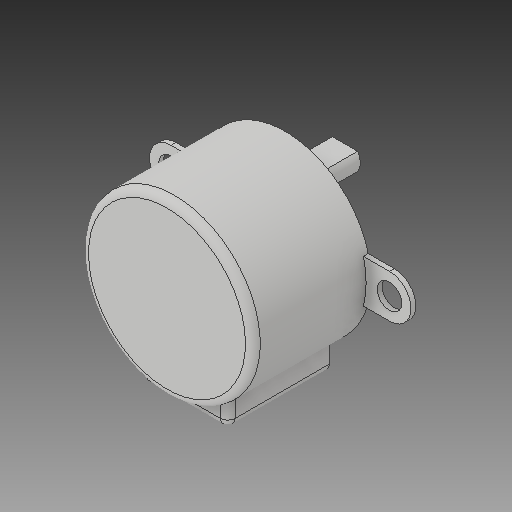
# Autodesk Inventor part: STEPPER MOTOR
Saved by Autodesk Inventor 2017 (Build 210142000, 142)
## iProperties
Created: 2017-04-01
Part Number: STEPPER MOTOR
Material: Generic
Document SubType Name: Modeling
Designer: Muchen
Density: 1 g/cm^3
Appearance: Default
Mass: 12.708 g
Surface Area: 34.3035 cm^2
Volume: 12.708 cm^3
Author: Muchen
Autodesk Inventor part; units mm, degrees
ref_plane "YZ Plane" through (0, 0, 0) normal (1, 0, 0) x (0, 1, 0)
ref_plane "XZ Plane" through (0, 0, 0) normal (0, 1, 0) x (-1, 0, 0)
ref_plane "XY Plane" through (0, 0, 0) normal (0, 0, 1) x (1, 0, 0)
sketch "Sketch1" plane through (0, 0, 0) normal (0, 0, 1) x (1, 0, 0)
  line L0 (0, 0) -> (0, 30.3704) construction
  line L1 (0, 0) -> (7.18, 0)
  line L2 (7.18, 0) -> (7.18, 4.46)
  arc A0 (0, 2.4704) -> (0, 30.3704) centre (0, 16.4204) ccw
  line L3 (13.5038, 19.9204) -> (17.75, 19.9204)
  arc A1 (17.75, 12.9204) -> (17.75, 19.9204) centre (17.75, 16.4204) ccw
  line L4 (17.75, 12.9204) -> (13.5038, 12.9204)
  circle A2 centre (17.75, 16.4204) radius 2
  line L5 (0, 0) -> (-7.18, 0)
  line L6 (-7.18, 0) -> (-7.18, 4.46)
  arc A3 (0, 30.3704) -> (0, 2.4704) centre (0, 16.4204) ccw
  line L7 (-13.5038, 19.9204) -> (-17.75, 19.9204)
  arc A4 (-17.75, 19.9204) -> (-17.75, 12.9204) centre (-17.75, 16.4204) ccw
  line L8 (-17.75, 12.9204) -> (-13.5038, 12.9204)
  circle A5 centre (-17.75, 16.4204) radius 2
  circle A6 centre (0, 22.2972) radius 4.61
  circle A7 centre (0, 22.2972) radius 2.5
  line L9 (2.0541, 23.7222) -> (-2.0541, 23.7222)
  line L10 (2.0541, 20.8722) -> (-2.0541, 20.8722)
  dimension "d0" = 13.95
  dimension "d1" = 7.18
  dimension "d2" = 4.46
  dimension "d3" = 3.5
  dimension "d4" = 4
  dimension "d11" = 9.22
  dimension "d12" = 5
  dimension "d13" = 2.85
  dimension "d26" = 35.5
  constraints: 22 end point, 18 point on circle, 8 centre point, 8 symmetric about line, 3 coincident, 3 parallel, 2 horizontal, 2 perpendicular, 2 point on line, 2 tangent, 1 horizontal alignment, 1 line through centre, 1 vertical, 3 other
  measures "d0" radius of A0
  measures "d1" distance of L0.start L1.end
  measures "d2" distance of L1.end L2.end
  measures "d3" radius of A1
  measures "d4" diameter of A2
  measures "d11" diameter of A6
  measures "d12" diameter of A7
  measures "d13" distance between parallel lines of L9 L10
  measures "d26" distance of A4.centre A2.centre
extrude "Extrusion1" add sketch "Sketch1" along normal blind 19.2 contours A0 A3 | A6 | A7 L10 L9 | L9 A7 | A7 L10
extrude "Extrusion2" add sketch "Sketch1" along normal blind 0.79 contours A0 L3 A1 L4 | L8 A4 L7 A3
extrude "Extrusion3" add sketch "Sketch1" along normal blind 16.5 contours L5 L6 A3 A0 L2 L1
extrude "Extrusion4" add sketch "Sketch1" against normal blind 1.75 contours A6
extrude "Extrusion5" add sketch "Sketch1" against normal blind 3.78 contours L9 A7 | A7 L10
extrude "Extrusion6" add sketch "Sketch1" against normal blind 9.73 contours A7 L10 L9
fillet "Fillet1" radius 1.2 6 edges at (7.18, 28.3807, 19.2) (7.18, 0, 8.25) (0, 0, 16.5) (-7.18, 0, 8.25) (-7.18, 2.23, 16.5) (7.18, 2.23, 16.5)
sketch "Sketch2" plane through (-5.98, 0, 0) normal (0, -1, 0) x (1, 0, 0)
  line L0 (8.98, 2.56) -> (2.98, 2.56) construction
  line L1 (8.98, 2) -> (2.98, 2)
  line L2 (2.98, 3.12) -> (8.98, 3.12)
  arc A0 (8.98, 2) -> (8.98, 3.12) centre (8.98, 2.56) ccw
  arc A1 (2.98, 3.12) -> (2.98, 2) centre (2.98, 2.56) ccw
  line L3 (0, 0) -> (11.96, 0) projected
  point P0 (5.98, 0)
  point P1 (5.98, 2.56)
  point P2 (5.98, 0)
  dimension "d21" = 2
  dimension "d22" = 1.12
  dimension "d23" = 6
  constraints: 8 end point, 4 point on circle, 4 tangent, 2 centre point, 2 midpoint, 1 horizontal, 1 parallel, 1 vertical alignment
  measures "d21" distance between parallel lines of L3 L1
  measures "d22" distance between parallel lines of L1 L2
  measures "d23" distance of L0.start L0.end
extrude "Extrusion7" cut sketch "Sketch2" against normal blind 2
body "Solid1"
